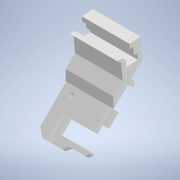
# Autodesk Inventor part: Button Holder
Saved by Autodesk Inventor 2020 (Build 240168000, 168)
## iProperties
Created: 2021-01-14
Part Number: Button Holder
Material: Generic
Document SubType Name: Sheet Metal
Designer: Luke
Density: 1 g/cm^3
Appearance: Default
Sheet Metal Rule: Default
Author: Luke
Autodesk Inventor part; units mm, degrees
ref_plane "YZ Plane" through (0, 0, 0) normal (1, 0, 0) x (0, 1, 0)
ref_plane "XZ Plane" through (0, 0, 0) normal (0, 1, 0) x (-1, 0, 0)
ref_plane "XY Plane" through (0, 0, 0) normal (0, 0, 1) x (1, 0, 0)
ref_plane "Work Plane3" through (59.9523, 18.4601, -23.7213) normal (0, -0.7071068, -0.7071068) x (1, 0, 0)
sketch "Sketch6" plane through (59.9523, 18.4601, -23.7213) normal (0, -0.7071068, -0.7071068) x (1, 0, 0)
  line L0 (-5.715, 11.43) -> (-6.985, 10.16) projected
  line L1 (-6.985, 10.16) -> (-6.985, -10.16) projected
  line L2 (-6.985, -10.16) -> (-5.715, -11.43) projected
  line L3 (-5.715, -11.43) -> (5.715, -11.43) projected
  line L4 (5.715, 11.43) -> (-5.715, 11.43) projected
  circle A0 centre (-5.08, 0) radius 0.9525 projected
  line L5 (6.985, 2.5) -> (-4.985, 2.5)
  line L6 (-4.985, -2.5) -> (6.985, -2.5)
  line L7 (6.985, -2.5) -> (6.985, 2.5)
  line L8 (-4.985, -10.02) -> (6.985, -10.02)
  line L9 (6.965, 10.18) -> (-4.985, 10.18)
  line L10 (-4.985, -10.02) -> (-4.985, -2.5)
  line L11 (-4.985, 2.5) -> (-4.985, 10.18)
  line L12 (7.2325, -10.4075) -> (5.86, -11.78)
  line L13 (5.86, -11.78) -> (-5.86, -11.78)
  line L14 (-5.86, -11.78) -> (-7.335, -10.305)
  line L15 (-7.335, -10.305) -> (-7.335, 10.305)
  line L16 (-7.335, 10.305) -> (-5.86, 11.78)
  line L17 (-5.86, 11.78) -> (5.86, 11.78)
  line L18 (5.86, 11.78) -> (7.2125, 10.4275)
  line L19 (6.985, -10.02) -> (6.985, -10.655)
  line L20 (6.965, 10.18) -> (6.965, 10.675)
  point P0 (-59.9523, 29.8267)
  point P1 (0, 0)
  dimension "d43" = 0.35
  constraints: 32 end point, 2 perpendicular, 2 point on line, 2 vertical, 1 horizontal, 1 parallel, 4 other
  measures "d43" distance between parallel lines of L3 L13
extrude "Extrusion5" add sketch "Sketch6" along normal blind 2
ref_plane "Work Plane5" through (59.9523, 19.3298, -22.8515) normal (0, 0.7071068, 0.7071068) x (-1, 0, 0)
sketch "Sketch7" plane through (59.9523, 19.3298, -22.8515) normal (0, 0.7071068, 0.7071068) x (-1, 0, 0)
  line L0 (4.985, 10.18) -> (-6.965, 10.18) projected
  line L1 (-6.965, 10.18) -> (-6.965, 10.675) projected
  line L2 (-6.965, 10.675) -> (-5.86, 11.78) projected
  line L3 (-5.86, 11.78) -> (5.86, 11.78) projected
  line L4 (5.86, 11.78) -> (7.335, 10.305) projected
  line L5 (7.335, 10.305) -> (7.335, -10.305) projected
  line L6 (7.335, -10.305) -> (5.86, -11.78) projected
  line L7 (5.86, -11.78) -> (-5.86, -11.78) projected
  line L8 (-5.86, -11.78) -> (-6.985, -10.655) projected
  line L9 (-6.985, -10.655) -> (-6.985, -10.02) projected
  line L10 (-6.985, -10.02) -> (4.985, -10.02) projected
  line L11 (4.985, -10.02) -> (4.985, -2.5) projected
  line L12 (4.985, -2.5) -> (-6.985, -2.5) projected
  line L13 (-6.985, -2.5) -> (-6.985, 2.5) projected
  line L14 (-6.985, 2.5) -> (4.985, 2.5) projected
  line L15 (4.985, 2.5) -> (4.985, 10.18) projected
  circle A0 centre (5.08, 0) radius 0.9525 projected
  line L16 (4.985, -2.5) -> (-6.985, -2.5) projected
  line L17 (4.985, -2.5) -> (-6.985, -2.5)
  line L18 (-6.985, -2.5) -> (-6.985, -5.25)
  line L19 (-6.985, -5.25) -> (4.985, -5.25)
  line L20 (4.985, -5.25) -> (4.985, -2.5)
  line L21 (4.985, 2.5) -> (-6.985, 2.5)
  line L22 (-6.985, 2.5) -> (-6.985, 5.25)
  line L23 (-6.985, 5.25) -> (4.985, 5.25)
  line L24 (4.985, 5.25) -> (4.985, 2.5)
  line L25 (4.985, -10.02) -> (4.985, -2.5) projected
  line L26 (4.985, -10.02) -> (-6.985, -10.02)
  line L27 (-6.985, -10.02) -> (-6.985, -7.29)
  line L28 (-6.985, -7.29) -> (4.985, -7.29)
  line L29 (4.985, -7.29) -> (4.985, -10.02)
  line L30 (4.985, 10.18) -> (4.985, 11.78)
  line L31 (-5.86, 11.78) -> (5.86, 11.78) projected
  point P0 (4.985, 5.25)
  point P1 (4.985, -7.29)
  point P2 (4.985, 11.78)
  dimension "d67" = 11.97
  dimension "d68" = 2.75
  dimension "d69" = 2.75
  constraints: 26 end point, 6 parallel, 4 perpendicular, 3 horizontal, 1 point on line
  measures "d67" distance of L19.end L18.end
  measures "d68" distance of L18.end L17.end
  measures "d69" distance of L21.end L22.end
extrude "Extrusion6" add sketch "Sketch7" along normal blind 2 contours L30 L3 L4 L5 L6 L7 L8 L9 L10 L11 L12 L13 L14 L15 | L15 L14 L22 L23 | L12 L11 L19 L18 | L11 L10 L27 L28
sketch "Sketch8" plane through (66.9373, 16.6923, -21.9535) normal (1, 0, 0) x (0, -0.7071068, -0.7071068)
  line L0 (0, 3.4525) -> (0, 1.5475) projected
  line L1 (0, 2.5) -> (-1.23, 2.5)
  line L2 (-1.23, 1.5475) -> (-1.23, 3.4525) projected
  line L3 (-1.315, 16.5647) -> (0.085, 16.5647)
  line L4 (0.085, 16.5647) -> (0.085, -11.5647)
  line L5 (0.085, -11.5647) -> (-1.315, -11.5647)
  line L6 (-1.315, -11.5647) -> (-1.315, 16.5647)
  line L7 (-1.315, 16.5647) -> (0.085, -11.5647) construction
  line L8 (0.085, 16.5647) -> (-1.315, -11.5647) construction
  point P0 (-3.7202, -27.3267)
  point P1 (-0.615, 2.5)
  dimension "d48" = 1.4
  constraints: 14 end point, 5 midpoint, 2 parallel, 1 horizontal, 1 perpendicular
  measures "d48" distance of L4.end L5.end
extrude "Extrusion7" cut sketch "Sketch8" against normal through all
sketch "Sketch9" plane through (59.9523, 17.0459, -25.1355) normal (0, -0.7071068, -0.7071068) x (-1, 0, 0)
  line L0 (0, -11.78) -> (5.86, -11.78)
  line L1 (5.86, -11.78) -> (7.335, -10.305) projected
  line L2 (7.335, -10.305) -> (7.335, 10.305) projected
  line L3 (7.335, 10.305) -> (5.86, 11.78) projected
  line L4 (5.86, 11.78) -> (0, 11.78)
  line L5 (1.5, 13.28) -> (6.4813, 13.28)
  line L6 (6.4813, 13.28) -> (8.835, 10.9263)
  line L7 (8.835, 10.9263) -> (8.835, -10.9263)
  line L8 (8.835, -10.9263) -> (6.4813, -13.28)
  line L9 (6.4813, -13.28) -> (1.5, -13.28)
  line L10 (-5.86, -11.78) -> (5.86, -11.78) projected
  line L11 (0, 11.78) -> (1.5, 13.28)
  line L12 (0, 11.78) -> (2.1213, 11.78) construction
  line L13 (0, -11.78) -> (1.5, -13.28)
  line L14 (0, -11.78) -> (2.1213, -11.78) construction
  point P0 (4.985, -10.18)
  dimension "d51" = 1.5
  dimension "d65" = 45
  dimension "d66" = 45
  constraints: 22 end point, 2 equal length, 2 horizontal, 2 other
  measures "d51" distance between parallel lines of L4 L5
  measures "d65" angle of L12 L11
  measures "d66" angle of L13 L14
extrude "Extrusion8" add sketch "Sketch9" against normal up to surface (5.23 mm away)
sketch "Sketch10" plane through (59.9523, 20.744, -21.4373) normal (0, 0.7071068, 0.7071068) x (1, 0, 0)
  line L0 (-1.5, -13.28) -> (-4.985, -13.28)
  line L1 (0, -11.78) -> (-1.5, -13.28)
  line L2 (-4.985, -11.78) -> (0, -11.78)
  line L3 (-4.985, -11.78) -> (0, -11.78) projected
  line L4 (-4.985, -11.78) -> (-4.985, -13.28)
  constraints: 8 end point, 1 perpendicular
extrude "Extrusion9" cut sketch "Sketch10" against normal up to surface (3.315 mm away)
ref_plane "Work Plane6" through (29.8053, 44.3484, 88.7721) normal (1, 0, 0) x (0, 1, 0)
ref_plane "Work Plane12" through (54.9673, 17.0459, -25.1355) normal (0, -0.7071068, 0.7071068) x (1, 0, 0)
ref_plane "Work Plane17" through (68.7248, 47.1761, -18.7491) normal (1, 0, 0) x (0, 0, -1)
sketch "Sketch20" plane through (68.7248, 47.1761, -18.7491) normal (1, 0, 0) x (0, 0, -1)
  line L0 (13.4196, -13.208) -> (9.2867, -13.5696)
  line L1 (9.2867, -13.5696) -> (9.0718, -11.1133)
  line L2 (9.0718, -11.1133) -> (7.5737, -9.8562)
  line L3 (7.5737, -9.8562) -> (7.1581, -9.8926)
  line L4 (15.0352, -14.0904) -> (14.3511, -6.2714)
  line L5 (14.3511, -6.2714) -> (10.3339, -6.6229)
  line L6 (10.3339, -6.6229) -> (10.4908, -8.4166)
  line L7 (10.4908, -8.4166) -> (11.7361, -8.3076)
  line L8 (11.7361, -8.3076) -> (11.9826, -11.1248)
  line L9 (11.9826, -11.1248) -> (13.2278, -11.0158)
  line L10 (13.2278, -11.0158) -> (13.4196, -13.208)
  line L11 (7.7881, -17.0933) -> (2.423, -22.4583)
  line L12 (2.423, -22.4583) -> (4.5451, -24.5804)
  line L13 (15.0352, -14.0904) -> (4.5451, -24.5804)
  line L14 (7.1581, -9.8926) -> (5.9129, -10.0015)
  line L15 (5.9129, -10.0015) -> (7.2671, -11.1378)
  line L16 (7.2671, -11.1378) -> (7.7881, -17.0933)
  point P0 (7.7881, -17.0933)
  constraints: 34 end point, 1 collinear
extrude "Extrusion13" add sketch "Sketch20" against normal up to surface (17.6076 mm away)
ref_plane "Work Plane23" through (59.921, 47.1761, -18.7491) normal (1, 0, 0) x (0, 0, -1)
chamfer "Chamfer7" distance 1.78 angle 45 7 edges at (62.8822, 29.0711, -29.7697) (59.2023, 29.6015, -30.3) (66.9373, 27.0859, -27.7845) (66.3747, 28.6734, -29.3719) (55.9616, 30.1318, -30.8303) (52.2941, 29.2996, -29.9982) (66.9373, 23.5247, -24.2233)
chamfer "Chamfer8" distance 2.75 angle 45 1 edges at (59.921, 24.7178, -21.1722)
body "Solid1"
